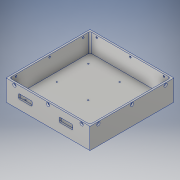
# Autodesk Inventor part: Housing_bottom
Saved by Autodesk Inventor 2018 (Build 220112000, 112)
## iProperties
Created: 2021-04-18
Part Number: Housing_bottom
Material: Aluminum 6061
Document SubType Name: Modeling
Designer: Ramana Bharathi
Density: 2.7 g/cm^3
Appearance: Aluminum - Flat
Mass: 1011.03 g
Surface Area: 1533.78 cm^2
Volume: 374.457 cm^3
Author: Ramana Bharathi
Autodesk Inventor part; units mm, degrees
note: some values were not read from the file. Chosen so that the rebuilt part matches the saved one: direction of "Hole2"; direction of "Hole3"; direction of "Hole4"; direction of "Hole5".
ref_plane "YZ Plane" through (0, 0, 0) normal (1, 0, 0) x (0, 1, 0)
ref_plane "XZ Plane" through (0, 0, 0) normal (0, 1, 0) x (-1, 0, 0)
ref_plane "XY Plane" through (0, 0, 0) normal (0, 0, 1) x (1, 0, 0)
sketch "Sketch1" plane through (0, 0, 0) normal (0, 1, 0) x (-1, 0, 0)
  line L0 (0, 0) -> (200, 0)
  line L1 (200, 0) -> (200, -200)
  line L2 (200, -200) -> (0, -200)
  line L3 (0, -200) -> (0, 0)
  dimension "d0" = 200
  dimension "d1" = 200
  constraints: 8 end point, 2 parallel, 1 horizontal, 1 perpendicular
  measures "d0" distance of L1.end L2.end
  measures "d1" distance of L0.end L1.end
extrude "Extrusion1" add sketch "Sketch1" along normal blind 50
sketch "Sketch2" plane through (0, 50, 0) normal (0, 1, 0) x (1, 0, 0)
  line L0 (-4, 4) -> (-196, 4)
  line L1 (-196, 4) -> (-196, 196)
  line L2 (-196, 196) -> (-4, 196)
  line L3 (-4, 196) -> (-4, 4)
  line L4 (-200, 0) -> (0, 0) projected
  line L5 (0, 0) -> (0, 200) projected
  dimension "d4" = 192
  dimension "d5" = 192
  dimension "d6" = 4
  dimension "d7" = 4
  constraints: 8 end point, 2 parallel, 1 horizontal, 1 perpendicular
  measures "d4" distance of L1.end L2.end
  measures "d5" distance of L0.end L1.end
  measures "d6" distance between parallel lines of L4 L0
  measures "d7" distance between parallel lines of L5 L3
extrude "Extrusion2" cut sketch "Sketch2" against normal blind 44
sketch "Sketch3" plane through (0, 6, 0) normal (0, 1, 0) x (1, 0, 0)
  line L0 (-185, 11) -> (-15, 11)
  line L1 (-15, 11) -> (-15, 181)
  line L2 (-15, 181) -> (-185, 181)
  line L3 (-185, 181) -> (-185, 11)
  line L4 (-196, 4) -> (-196, 196) projected
  line L5 (-4, 4) -> (-196, 4) projected
  circle A0 centre (-175, 171) radius 1.5
  circle A1 centre (-175, 96) radius 1.5
  circle A2 centre (-175, 21) radius 1.5
  circle A3 centre (-100, 171) radius 1.5
  circle A4 centre (-100, 96) radius 1.5
  circle A5 centre (-100, 21) radius 1.5
  circle A6 centre (-25, 171) radius 1.5
  circle A7 centre (-25, 96) radius 1.5
  circle A8 centre (-25, 21) radius 1.5
  point P0 (0, 0)
  dimension "d10" = 170
  dimension "d11" = 170
  dimension "d12" = 11
  dimension "d13" = 7
  dimension "d14" = 3
  dimension "d15" = 10
  dimension "d16" = 10
  dimension "d19" = 75
  dimension "d22" = 75
  constraints: 9 centre point, 8 end point, 2 horizontal, 2 parallel, 1 perpendicular, 1 vertical, 16 other
  measures "d10" distance of L2.end L1.end
  measures "d11" distance of L1.end L0.end
  measures "d12" distance between parallel lines of L4 L3
  measures "d13" distance between parallel lines of L5 L0
  measures "d14" diameter of A0
  measures "d15" distance from line of L2 A0.centre
  measures "d16" distance from line of A0.centre L3
  measures "d19" distance of A0.centre A1.centre
  measures "d22" distance of A0.centre A3.centre
sketch "Sketch4" plane through (0, 0, 0) normal (1, 0, 0) x (0, 0, -1)
  circle A0 centre (20, 45) radius 2
  line L0 (0, 50) -> (200, 50) projected
  line L1 (0, 0) -> (0, 50) projected
  circle A1 centre (100, 45) radius 2
  circle A2 centre (180, 45) radius 2
  dimension "d25" = 4
  dimension "d27" = 5
  dimension "d29" = 20
  dimension "d32" = 80
  constraints: 3 centre point, 1 horizontal, 4 other
  measures "d25" diameter of A0
  measures "d27" distance from line of L0 A0.centre
  measures "d29" distance from line of L1 A0.centre
  measures "d32" distance of A0.centre A1.centre
sketch "Sketch5" plane through (-200, 0, 0) normal (0, 0, 1) x (1, 0, 0)
  circle A0 centre (20, 45) radius 2
  line L0 (0, 50) -> (200, 50) projected
  line L1 (0, 0) -> (0, 50) projected
  circle A1 centre (100, 45) radius 2
  circle A2 centre (180, 45) radius 2
  point P0 (200, 0)
  dimension "d43" = 4
  dimension "d44" = 5
  dimension "d45" = 20
  dimension "d48" = 80
  constraints: 3 centre point, 1 horizontal, 4 other
  measures "d43" diameter of A0
  measures "d44" distance from line of L0 A0.centre
  measures "d45" distance from line of L1 A0.centre
  measures "d48" distance of A0.centre A1.centre
fillet "Fillet1" radius 4 4 edges at (-196, 28, -196) (-196, 28, -4) (-4, 28, -4) (-4, 28, -196)
sketch "Sketch7" plane through (-200, 0, 0) normal (0, 0, 1) x (1, 0, 0)
  line L0 (30, 22) -> (62, 22)
  line L1 (62, 22) -> (62, 33)
  line L2 (62, 33) -> (30, 33)
  line L3 (30, 33) -> (30, 22)
  line L4 (127, 22) -> (159, 22)
  line L5 (159, 22) -> (159, 33)
  line L6 (159, 33) -> (127, 33)
  line L7 (127, 33) -> (127, 22)
  line L8 (0, 0) -> (0, 50) projected
  line L9 (200, 0) -> (0, 0) projected
  dimension "d114" = 32
  dimension "d115" = 11
  dimension "d116" = 32
  dimension "d117" = 11
  dimension "d121" = 65
  dimension "d122" = 30
  dimension "d123" = 22
  dimension "d124" = 22
  constraints: 16 end point, 4 parallel, 2 horizontal, 2 perpendicular
  measures "d114" distance of L2.end L1.end
  measures "d115" distance of L1.end L0.end
  measures "d116" distance of L6.end L5.end
  measures "d117" distance of L5.end L4.end
  measures "d121" distance between parallel lines of L7 L1
  measures "d122" distance between parallel lines of L8 L3
  measures "d123" distance between parallel lines of L9 L0
  measures "d124" distance between parallel lines of L9 L4
extrude "Extrusion8" cut sketch "Sketch7" against normal up to surface (4 mm away)
hole "Hole1" at (-100, 6, -96) at (-175, 6, -96) at (-175, 6, -21) at (-100, 6, -21) at (-175, 6, -171) at (-100, 6, -171) at (-25, 6, -171) at (-25, 6, -96) at (-25, 6, -21) direction (0, -1, 0) diameter 3 depth 5 tip angle 118
hole "Hole2" at (0, 45, -20) at (0, 45, -100) at (0, 45, -180) direction (-1, 0, 0) diameter 4 end up to surface countersink diameter 8 countersink angle 90
hole "Hole3" at (-20, 45, 0) at (-100, 45, 0) at (-180, 45, 0) direction (0, 0, -1) diameter 4 end up to surface countersink diameter 8 countersink angle 90
sketch "Sketch8" plane through (-200, 0, -200) normal (-1, 0, 0) x (0, 0, 1)
  circle A0 centre (20, 45) radius 2
  line L0 (0, 50) -> (200, 50)
  line L1 (0, 0) -> (0, 50)
  circle A1 centre (100, 45) radius 2
  circle A2 centre (180, 45) radius 2
  point P0 (200, 0)
  dimension "d172" = 4
  dimension "d173" = 5
  dimension "d174" = 20
  dimension "d175" = 80
  constraints: 4 end point, 3 centre point, 1 horizontal, 4 other
  measures "d172" diameter of A0
  measures "d173" distance from line of L0 A0.centre
  measures "d174" distance from line of L1 A0.centre
  measures "d175" distance of A0.centre A1.centre
hole "Hole4" at (-200, 45, -180) at (-200, 45, -100) at (-200, 45, -20) direction (1, 0, 0) diameter 4 end up to surface countersink diameter 8 countersink angle 90
sketch "Sketch9" plane through (0, 0, -200) normal (0, 0, -1) x (-1, 0, 0)
  circle A0 centre (20, 45) radius 2
  line L0 (0, 50) -> (200, 50)
  line L1 (0, 0) -> (0, 50)
  circle A1 centre (100, 45) radius 2
  circle A2 centre (180, 45) radius 2
  circle A3 centre (20, 45) radius 2
  line L2 (0, 50) -> (200, 50)
  line L3 (0, 0) -> (0, 50)
  circle A4 centre (100, 45) radius 2
  circle A5 centre (180, 45) radius 2
  circle A6 centre (20, 45) radius 2
  line L4 (0, 50) -> (200, 50)
  line L5 (0, 0) -> (0, 50)
  circle A7 centre (100, 45) radius 2
  circle A8 centre (180, 45) radius 2
  dimension "d188" = 4
  dimension "d189" = 5
  dimension "d190" = 20
  dimension "d191" = 80
  dimension "d197" = 4
  dimension "d198" = 5
  dimension "d199" = 20
  dimension "d200" = 80
  dimension "d206" = 4
  dimension "d207" = 5
  dimension "d208" = 20
  dimension "d209" = 80
  constraints: 12 end point, 9 centre point, 3 horizontal, 12 other
  measures "d188" diameter of A0
  measures "d189" distance from line of L0 A0.centre
  measures "d190" distance from line of L1 A0.centre
  measures "d191" distance of A0.centre A1.centre
  measures "d197" diameter of A3
  measures "d198" distance from line of L2 A3.centre
  measures "d199" distance from line of L3 A3.centre
  measures "d200" distance of A3.centre A4.centre
  measures "d206" diameter of A6
  measures "d207" distance from line of L4 A6.centre
  measures "d208" distance from line of L5 A6.centre
  measures "d209" distance of A6.centre A7.centre
hole "Hole5" at (-20, 45, -200) at (-100, 45, -200) at (-180, 45, -200) direction (0, 0, 1) diameter 4 end up to surface countersink diameter 8 countersink angle 90
thread "Thread25" size "M3x0.5" class "6H" standard "ANSI Metric M Profile" full length
thread "Thread26" size "M3x0.5" class "6H" standard "ANSI Metric M Profile" full length
thread "Thread27" size "M3x0.5" class "6H" standard "ANSI Metric M Profile" full length
thread "Thread28" size "M3x0.5" class "6H" standard "ANSI Metric M Profile" full length
thread "Thread29" size "M3x0.5" class "6H" standard "ANSI Metric M Profile" full length
thread "Thread30" size "M3x0.5" class "6H" standard "ANSI Metric M Profile" full length
thread "Thread31" size "M3x0.5" class "6H" standard "ANSI Metric M Profile" full length
thread "Thread32" size "M3x0.5" class "6H" standard "ANSI Metric M Profile" full length
thread "Thread33" size "M3x0.5" class "6H" standard "ANSI Metric M Profile" full length
thread "Thread34" size "M4x0.7" class "6H" standard "ANSI Metric M Profile" full length
thread "Thread35" size "M4x0.7" class "6H" standard "ANSI Metric M Profile" full length
thread "Thread36" size "M4x0.7" class "6H" standard "ANSI Metric M Profile" full length
thread "Thread37" size "M4x0.7" class "6H" standard "ANSI Metric M Profile" full length
thread "Thread38" size "M4x0.7" class "6H" standard "ANSI Metric M Profile" full length
thread "Thread39" size "M4x0.7" class "6H" standard "ANSI Metric M Profile" full length
thread "Thread40" size "M4x0.7" class "6H" standard "ANSI Metric M Profile" full length
thread "Thread41" size "M4x0.7" class "6H" standard "ANSI Metric M Profile" full length
thread "Thread42" size "M4x0.7" class "6H" standard "ANSI Metric M Profile" full length
thread "Thread43" size "M4x0.7" class "6H" standard "ANSI Metric M Profile" full length
thread "Thread44" size "M4x0.7" class "6H" standard "ANSI Metric M Profile" full length
thread "Thread45" size "M4x0.7" class "6H" standard "ANSI Metric M Profile" full length
fillet "Fillet2" radius 2 8 edges at (-170, 22, -2) (-138, 33, -2) (-138, 22, -2) (-170, 33, -2) (-41, 33, -2) (-73, 33, -2) (-73, 22, -2) (-41, 22, -2)
body "Solid1"
